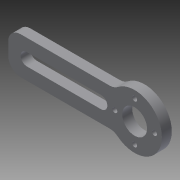
# Autodesk Inventor part: moving_arm
Saved by Autodesk Inventor 2014 (Build 180170000, 170)
## iProperties
Created: 2014-01-12
Part Number: moving_arm
Material: Générique
Document SubType Name: Modeling
Designer: helly
Density: 1 g/cm^3
Appearance: Par défaut
Author: helly
Autodesk Inventor part; units mm, degrees
ref_plane "YZ Plane" through (0, 0, 0) normal (1, 0, 0) x (0, 1, 0)
ref_plane "XZ Plane" through (0, 0, 0) normal (0, 1, 0) x (-1, 0, 0)
ref_plane "XY Plane" through (0, 0, 0) normal (0, 0, 1) x (1, 0, 0)
sketch "Esquisse1" plane through (0, 0, 0) normal (0, 1, 0) x (-1, 0, 0)
  circle A0 centre (8, 0) radius 1
  circle A1 centre (0, 8) radius 1
  circle A2 centre (-8, 0) radius 1
  circle A3 centre (0, -8) radius 1
  line L0 (0, 0) -> (-8, 0) construction
  circle A4 centre (0, 0) radius 11 construction
  line L1 (0, 0) -> (77, 0) construction
  line L2 (0, 0) -> (0, 2.5) construction
  line L3 (0, 2.5) -> (0, 7.5) construction
  line L4 (0, 7.5) -> (8.0467, 7.5) construction
  line L5 (0, 2.5) -> (10.7121, 2.5) construction
  line L6 (11, 0) -> (46, 0) construction
  line L7 (46, 0) -> (51, 0) construction
  line L8 (8.0467, 7.5) -> (51, 7.5)
  line L9 (51, 7.5) -> (51, 0)
  line L10 (10.7121, 2.5) -> (46, 2.5) construction
  line L11 (46, 2.5) -> (46, 0) construction
  line L12 (11, 0) -> (11, 2.5) construction
  arc A5 (8.0467, 7.5) -> (-11, 0) centre (0, 0) ccw
  line L13 (11, 0) -> (13.5, 0) construction
  line L14 (46, 0) -> (43.5, 0) construction
  arc A6 (13.5, 2.5) -> (11, 0) centre (13.5, 0) ccw
  arc A7 (46, 0) -> (43.5, 2.5) centre (43.5, 0) ccw
  line L15 (13.5, 2.5) -> (43.5, 2.5)
  line L16 (8.0467, -7.5) -> (51, -7.5)
  line L17 (51, -7.5) -> (51, 0)
  arc A8 (-11, 0) -> (8.0467, -7.5) centre (0, 0) ccw
  arc A9 (11, 0) -> (13.5, -2.5) centre (13.5, 0) ccw
  arc A10 (43.5, -2.5) -> (46, 0) centre (43.5, 0) ccw
  line L18 (13.5, -2.5) -> (43.5, -2.5)
  circle A11 centre (0, 0) radius 5
  dimension "d7" = 360
  dimension "d12" = 2
  dimension "d13" = 8
  dimension "d14" = 22
  dimension "d19" = 2.5
  dimension "d20" = 5
  dimension "d21" = 35
  dimension "d22" = 5
  dimension "d29" = 10
  constraints: 38 end point, 15 point on circle, 12 centre point, 8 perpendicular, 6 point on line, 5 coincident, 4 symmetric about line, 3 collinear, 3 tangent, 2 parallel, 1 concentric, 1 horizontal, 12 other
  measures "d12" diameter of A0
  measures "d13" distance of L0.start L0.end
  measures "d14" diameter of A4
  measures "d19" distance of L1.start L2.end
  measures "d20" distance of L2.end L3.end
  measures "d21" distance of L6.start L6.end
  measures "d22" distance of L6.end L7.end
  measures "d29" diameter of A11
extrude "Extrusion2" add sketch "Esquisse1" along normal blind 4
fillet "Congé5" radius 5 1 edges at (-51, 2, 7.5)
fillet "Congé6" radius 5 1 edges at (-51, 2, -7.5)
fillet "Congé7" radius 5 1 edges at (-8.0467, 2, 7.5)
fillet "Congé8" radius 5 1 edges at (-8.0467, 2, -7.5)
